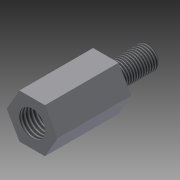
# Autodesk Inventor part: spacer1cm
Saved by Autodesk Inventor 2015 (Build 190159000, 159)
## iProperties
Created: 2015-01-19
Part Number: spacer1cm
Material: Generic
Document SubType Name: Modeling
Designer: Rafi Kurnia Putra
Density: 1 g/cm^3
Appearance: Default
Mass: 0.294333 g
Surface Area: 3.89895 cm^2
Volume: 0.294333 cm^3
Author: Rafi Kurnia Putra
Autodesk Inventor part; units mm, degrees
ref_plane "YZ Plane" through (0, 0, 0) normal (1, 0, 0) x (0, 1, 0)
ref_plane "XZ Plane" through (0, 0, 0) normal (0, 1, 0) x (-1, 0, 0)
ref_plane "XY Plane" through (0, 0, 0) normal (0, 0, 1) x (1, 0, 0)
sketch "Sketch1" plane through (0, 0, 0) normal (0, 1, 0) x (-1, 0, 0)
  line L0 (-3.4641, 0) -> (-1.7321, 3)
  line L1 (-1.7321, 3) -> (1.7321, 3)
  line L2 (1.7321, 3) -> (3.4641, 0)
  line L3 (3.4641, 0) -> (1.7321, -3)
  line L4 (1.7321, -3) -> (-1.7321, -3)
  line L5 (-1.7321, -3) -> (-3.4641, 0)
  point P0 (0, 0)
  point P1 (0, 0)
  dimension "d1" = 6
  constraints: 12 end point, 1 coincident, 13 other
  measures "d1" distance between parallel lines of L4 L1
extrude "Extrusion1" add sketch "Sketch1" along normal blind 10
sketch "Sketch2" plane through (0, 0, 0) normal (0, -1, 0) x (1, 0, 0)
  circle A0 centre (0, 0) radius 1.75
  dimension "d4" = 3.5
  constraints: 1 centre point, 1 coincident
  measures "d4" diameter of A0
sketch "Sketch3" plane through (0, 10, 0) normal (0, 1, 0) x (1, 0, 0)
  circle A0 centre (0, 0) radius 1.5
  dimension "d5" = 3
  constraints: 1 centre point, 1 coincident
  measures "d5" diameter of A0
extrude "Extrusion2" add sketch "Sketch3" along normal blind 5.7
extrude "Extrusion3" cut sketch "Sketch2" against normal blind 6
thread "Thread1" size "M3x0.35" class "6g" standard "ANSI Metric M Profile" full length
thread "Thread2" size "M4x0.5" class "6H" standard "ANSI Metric M Profile" full length
body "Solid1"
